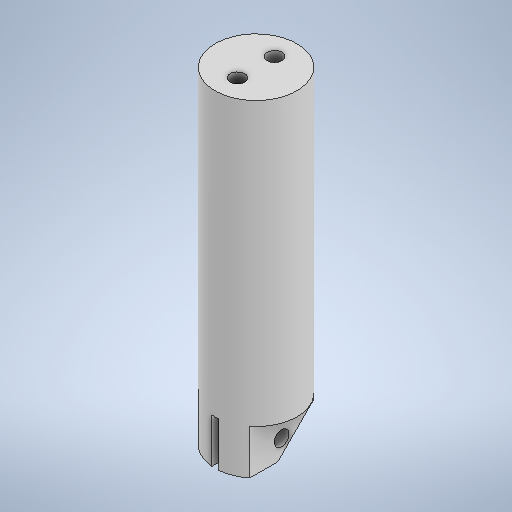
# Autodesk Inventor part: Part4 finger(index)
Saved by Autodesk Inventor 2025 (Build 290162000, 162)
## iProperties
Created: 2025-10-18
Part Number: Part4 finger(index)
Material: Generic
Document SubType Name: Modeling
Designer: abdul
Density: 1 g/cm^3
Appearance: Default
Author: abdul
Autodesk Inventor part; units mm, degrees
ref_plane "YZ Plane" through (0, 0, 0) normal (1, 0, 0) x (0, 1, 0)
ref_plane "XZ Plane" through (0, 0, 0) normal (0, 1, 0) x (-1, 0, 0)
ref_plane "XY Plane" through (0, 0, 0) normal (0, 0, 1) x (1, 0, 0)
sketch "Sketch1" plane through (0, 0, 0) normal (0, 1, 0) x (-1, 0, 0)
  circle A0 centre (0, 0) radius 5.5
  dimension "d0" = 11
  constraints: 1 centre point, 1 coincident
  measures "d0" diameter of A0
extrude "Extrusion1" add sketch "Sketch1" along normal blind 38
sketch "Sketch6" plane through (0, 0, 0) normal (0, -1, 0) x (1, 0, 0)
  circle A0 centre (0, 0) radius 5.5 projected
  line L0 (3.45, 0) -> (3.45, -4.2834)
  line L1 (0.45, 0) -> (0.45, -5.4816)
  line L2 (3.45, -5.4816) -> (3.45, -4.2834)
  line L3 (3.45, -5.4816) -> (0.45, -5.4816)
  line L4 (0.45, 0) -> (0.45, 5.4816)
  line L5 (3.45, 5.3243) -> (3.45, 0)
  line L6 (3.45, 5.3243) -> (0.45, 5.4816)
  line L7 (0, -5.5) -> (0, 5.5)
  line L8 (-3.45, 0) -> (-3.45, -4.2834)
  line L9 (-0.45, 0) -> (-0.45, -5.4816)
  line L10 (-3.45, -5.4816) -> (-3.45, -4.2834)
  line L11 (-3.45, -5.4816) -> (-0.45, -5.4816)
  line L12 (-0.45, 0) -> (-0.45, 5.4816)
  line L13 (-3.45, 5.3243) -> (-3.45, 0)
  line L14 (-3.45, 5.3243) -> (-0.45, 5.4816)
  point P0 (-3.45, 4.2834)
  point P1 (3.45, 4.2834)
  dimension "d20" = 3
  dimension "d21" = 3
  dimension "d22" = 0.45
  dimension "d23" = 2.05
  dimension "d24" = 2.05
  constraints: 30 end point, 7 symmetric about line, 5 point on circle, 4 point on line, 3 parallel, 1 perpendicular, 1 vertical
  measures "d20" distance of L0.start L1.start
  measures "d21" angle of L3 L6
  measures "d22" distance from line of point (0, 0) L1
  measures "d23" distance edge to line of A0 L0
  measures "d24" distance edge to line of A0 L8
extrude "Extrusion5" add sketch "Sketch6" along normal blind 6 contours A0 L5 L0 L1 L4 | L12 L9 A0 L8 L13
sketch "Sketch8" plane through (0, 0, 0) normal (1, 0, 0) x (0, 1, 0)
  line L0 (0, -5.5) -> (38, -5.5) projected
  line L1 (0, -5.4816) -> (-6, -5.4816) projected
  line L2 (0, -5.4816) -> (0, 5.4816) projected
  line L3 (0, -5.4816) -> (-6, 0.5184)
  line L4 (0, -5.4816) -> (8.4853, -5.4816) construction
  line L5 (-6, -5.4816) -> (-6, 5.4816) projected
  line L6 (-6, 0.5184) -> (-6, -5.4816)
  point P0 (0, 0)
  dimension "d27" = 135
  constraints: 6 end point, 1 equal length, 1 horizontal, 1 perpendicular, 1 point on line
  measures "d27" angle of L4 L3
extrude "Extrusion6" cut sketch "Sketch8" along normal through all both and the other way through all
sketch "Sketch10" plane through (0, 0, 0) normal (1, 0, 0) x (0, 1, 0)
  circle A0 centre (-3.5, 0) radius 1
  line L0 (0, -5.5) -> (38, -5.5) projected
  line L1 (-6, 0.5184) -> (-6, 5.4816) projected
  point P0 (0, 0)
  dimension "d30" = 2
  dimension "d31" = 5.5
  dimension "d32" = 2.5
  constraints: 1 centre point
  measures "d30" diameter of A0
  measures "d31" distance from line of A0.centre L0
  measures "d32" distance from line of A0.centre L1
extrude "Extrusion7" cut sketch "Sketch10" along normal through all both and the other way through all
sketch "Sketch11" plane through (0, 38, 0) normal (0, 1, 0) x (1, 0, 0)
  circle A0 centre (0, 2.5) radius 1
  circle A1 centre (0, -2.5) radius 1
  point P0 (0, 0)
  dimension "d35" = 2
  dimension "d36" = 2
  dimension "d37" = 2.5
  dimension "d38" = 2.5
  constraints: 2 centre point
  measures "d35" diameter of A0
  measures "d36" diameter of A1
  measures "d37" distance of point (0, 0) A0.centre
  measures "d38" distance of point (0, 0) A1.centre
extrude "Extrusion8" cut sketch "Sketch11" against normal blind 38
body "Solid1"
